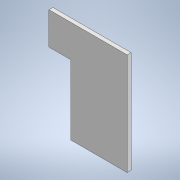
# Autodesk Inventor part: PCB_2_Miras
Saved by Autodesk Inventor 2022 (Build 260153000, 153)
## iProperties
Created: 2023-01-03
Part Number: PCB_2_Miras
Material: Generic
Document SubType Name: Modeling
Designer: Kamil
Density: 1 g/cm^3
Appearance: Default
Author: Kamil
Autodesk Inventor part; units mm, degrees
ref_plane "YZ Plane" through (0, 0, 0) normal (1, 0, 0) x (0, 1, 0)
ref_plane "XZ Plane" through (0, 0, 0) normal (0, 1, 0) x (-1, 0, 0)
ref_plane "XY Plane" through (0, 0, 0) normal (0, 0, 1) x (1, 0, 0)
sketch "Sketch1" plane through (0, 0, 0) normal (0, 0, 1) x (1, 0, 0)
  line L0 (12.5, -5.24) -> (15, -5.24) projected
  line L1 (15, -5.24) -> (15, -10.24) projected
  line L2 (15, -10.24) -> (12.5, -10.24) projected
  arc A0 (12.5, -5.24) -> (12.5, -10.24) centre (12.5, -7.74) ccw projected
  line L3 (-15, -5.24) -> (-12.5, -5.24) projected
  arc A1 (-12.5, -10.24) -> (-12.5, -5.24) centre (-12.5, -7.74) ccw projected
  line L4 (-12.5, -10.24) -> (-15, -10.24) projected
  line L5 (-15, -10.24) -> (-15, -5.24) projected
  circle A2 centre (-7.5, -12.2) radius 1.75 projected
  circle A3 centre (7.5, -12.2) radius 1.75 projected
  line L6 (37.5, 31.0066) -> (-37.5, 31.0066) projected
  line L7 (-37.5, 31.0066) -> (-37.5, -15.4) projected
  line L8 (-37.5, -15.4) -> (37.5, -15.4) projected
  line L9 (37.5, -15.4) -> (37.5, -10.4) projected
  line L10 (17.8602, 13.1005) -> (17.8602, -3.2) projected
  line L11 (17.8602, -3.2) -> (11.3436, -3.2) projected
  line L12 (11.3436, -3.2) -> (6.7283, -5.8186) projected
  line L13 (6.7283, -5.8186) -> (-6.7283, -5.8186) projected
  line L14 (-6.7283, -5.8186) -> (-11.3436, -3.2) projected
  line L15 (-11.3436, -3.2) -> (-17.8602, -3.2) projected
  line L16 (-17.8602, -3.2) -> (-17.8602, 13.1005) projected
  line L17 (-13.55, 13.1005) -> (-17.8602, 13.1005) projected
  line L18 (-13.55, 23.254) -> (-13.55, 13.1005) projected
  line L19 (2.4, 23.254) -> (-13.55, 23.254) projected
  line L20 (2.4, 25.954) -> (2.4, 23.254) projected
  line L21 (4, 25.954) -> (2.4, 25.954) projected
  line L22 (4, 23.254) -> (4, 25.954) projected
  line L23 (8.95, 23.254) -> (4, 23.254) projected
  line L24 (8.95, 13.1005) -> (8.95, 23.254) projected
  line L25 (17.8602, 13.1005) -> (8.95, 13.1005) projected
  line L26 (50, 22.6643) -> (44, 22.6643) projected
  line L27 (44, 22.6643) -> (44, -4.7413) projected
  arc A4 (44, -9.7413) -> (44, -4.7413) centre (44, -7.2413) ccw projected
  line L28 (44, -9.7413) -> (44, -18.8012) projected
  line L29 (44, -18.8012) -> (50, -18.8012) projected
  line L30 (50, -18.8012) -> (50, 22.6643) projected
  line L31 (40.2471, -8.6254) -> (44, -18.8012) projected
  line L32 (44, -9.7413) -> (44, -18.8012) projected
  arc A5 (44, -4.7413) -> (44, -9.7413) centre (44, -7.2413) ccw projected
  line L33 (44, 4.3187) -> (44, -4.7413) projected
  line L34 (44, 4.3187) -> (40.2471, -5.8572) projected
  arc A6 (40.2471, -5.8572) -> (40.2471, -8.6254) centre (44, -7.2413) ccw projected
  line L35 (8.95, 13.1005) -> (37.5, 13.1005)
  line L36 (37.5, 13.1005) -> (37.5, 31.0066)
  line L37 (37.5, 31.0066) -> (8.95, 31.0066)
  line L38 (8.95, 31.0066) -> (8.95, 13.1005)
  line L39 (44, 18.1772) -> (41, 18.1772)
  line L40 (41, 18.1772) -> (41, 7.8033)
  line L41 (41, 7.8033) -> (44, 7.8033)
  line L42 (44, 7.8033) -> (44, 18.1772)
  line L43 (37.5, 31.0066) -> (41, 31.0066)
  line L44 (41, 31.0066) -> (41, 1.9316)
  line L45 (41, 1.9316) -> (37.5, 1.9316)
  line L46 (37.5, 1.9316) -> (37.5, 31.0066)
  line L47 (8.95, 31.0066) -> (41, 31.0066)
  line L48 (41, 31.0066) -> (41, 23.254)
  line L49 (41, 23.254) -> (8.95, 23.254)
  line L50 (8.95, 23.254) -> (8.95, 31.0066)
  line L51 (17.8602, 13.1005) -> (37.5, 13.1005)
  line L52 (37.5, 13.1005) -> (37.5, -15.4)
  line L53 (37.5, -15.4) -> (17.8602, -15.4)
  line L54 (17.8602, -15.4) -> (17.8602, 13.1005)
  line L55 (37.5, -15.4) -> (41, -15.4)
  line L56 (41, -15.4) -> (41, 1.9316)
  line L57 (41, 1.9316) -> (37.5, 1.9316)
  line L58 (37.5, 1.9316) -> (37.5, -15.4)
  circle A7 centre (36, -10.4) radius 1.5 projected
  line L59 (37.5, -10.4) -> (37.5, 31.0066) projected
  arc A8 (-17.7252, -6.9095) -> (-17.704, -4.5096) centre (-17.7146, -5.7096) ccw projected
  line L60 (-17.7252, -6.9095) -> (-18.8252, -6.8998) projected
  arc A9 (-18.8039, -4.4999) -> (-18.8252, -6.8998) centre (-18.8145, -5.6998) ccw projected
  line L61 (-18.8039, -4.4999) -> (-17.704, -4.5096) projected
  circle A10 centre (21.3634, 8.1005) radius 1.5 projected
  arc A11 (-17.5172, 16.5895) -> (-17.496, 18.9894) centre (-17.5066, 17.7895) ccw projected
  line L62 (-17.5172, 16.5895) -> (-18.6172, 16.5993) projected
  arc A12 (-18.5959, 18.9992) -> (-18.6172, 16.5993) centre (-18.6065, 17.7992) ccw projected
  line L63 (-18.5959, 18.9992) -> (-17.496, 18.9894) projected
  point P0 (0, 0)
  point P1 (41, -3.8157)
  point P2 (8.95, 31.0066)
  point P3 (41, -10.6668)
  dimension "d0" = 3
  constraints: 48 end point, 12 parallel, 6 horizontal, 6 perpendicular, 2 point on line, 1 horizontal alignment
  measures "d0" distance of L41.end L40.end
extrude "Extrusion1" add sketch "Sketch1" along normal blind 3.1 contours L36 L49 L38 L6 | L43 L44 L49 L36 | L49 L44 L40 L45 L46 L36 | L36 L35 L25 L24 L49 | A7 | L46 L52 L9 L8 L54 L10 L35 | L45 L56 L34 A6 L31 L55 L9 L52 | A10
sketch "Sketch2" plane through (0, 0, 0) normal (0, 0, -1) x (-1, 0, 0)
  line L0 (-40.2471, -5.8572) -> (-41, -3.8157) projected
  arc A0 (-40.2471, -8.6254) -> (-40.2471, -5.8572) centre (-44, -7.2413) ccw projected
  line L1 (-41, -10.6668) -> (-40.2471, -8.6254) projected
  line L2 (-41, -15.4) -> (-41, -10.6668) projected
  line L3 (-17.8602, -15.4) -> (-41, -15.4) projected
  line L4 (-17.8602, 13.1005) -> (-17.8602, -15.4) projected
  line L5 (-8.95, 13.1005) -> (-17.8602, 13.1005) projected
  line L6 (-8.95, 31.0066) -> (-8.95, 13.1005) projected
  line L7 (-41, 31.0066) -> (-8.95, 31.0066) projected
  line L8 (-41, -3.8157) -> (-41, 31.0066) projected
  point P0 (0, 0)
extrude "Extrusion2" cut sketch "Sketch2" against normal blind 1.5
sketch "Sketch3" plane through (41, -3.8157, 3.1) normal (1, 0, 0) x (0, 0, -1)
  line L0 (24.6867, 44.1065) -> (27.0867, 44.1065) projected
  line L1 (27.0867, 44.1065) -> (27.0867, 31.3518) projected
  line L2 (27.0867, 31.3518) -> (24.6867, 31.3518) projected
  line L3 (24.6867, 31.3518) -> (24.6867, 44.1065) projected
  line L4 (36.2, 74.2694) -> (-3.9, 26.48) projected
  line L5 (-3.9, -14.9855) -> (-3.9, 26.48) projected
  line L6 (-3.9, -14.9855) -> (7.1, -14.9855) projected
  line L7 (7.1, -14.9855) -> (7.1, 1.1145) projected
  arc A0 (25.2, 19.2145) -> (7.1, 1.1145) centre (25.2, 1.1145) ccw projected
  line L8 (25.2, 19.2145) -> (36.2, 19.2145) projected
  line L9 (36.2, 19.2145) -> (36.2, 74.2694) projected
  line L10 (1.6, 0) -> (1.6, 34.8223) projected
  line L11 (1.6, 34.8223) -> (0, 34.8223) projected
  line L12 (0, 0) -> (0, 34.8223) projected
  line L13 (1.6, 0) -> (0, 0) projected
  line L14 (0, 0) -> (0, 34.8223) projected
  line L15 (0, 30.197) -> (1.6, 30.197)
  point P0 (3.1, 3.8157)
  constraints: 2 end point, 2 point on line, 1 perpendicular
extrude "Extrusion3" cut sketch "Sketch3" against normal through all contours L10 L15 L12 L4 | L4 L12 L11 L10
sketch "Sketch4" plane through (0, 0, 3.1) normal (0, 0, 1) x (1, 0, 0)
  line L0 (31.7, -15.7) -> (31.7, 9.3) projected
  line L1 (41, 26.3813) -> (8.95, 26.3813) projected
  line L2 (8.95, 26.3813) -> (8.95, 13.1005) projected
  line L3 (8.95, 13.1005) -> (17.8602, 13.1005) projected
  line L4 (17.8602, 13.1005) -> (17.8602, -15.4) projected
  line L5 (17.8602, -15.4) -> (41, -15.4) projected
  line L6 (41, -15.4) -> (41, -10.6668) projected
  line L7 (41, -10.6668) -> (40.2471, -8.6254) projected
  arc A0 (40.2471, -5.8572) -> (40.2471, -8.6254) centre (44, -7.2413) ccw projected
  line L8 (40.2471, -5.8572) -> (41, -3.8157) projected
  line L9 (41, -3.8157) -> (41, 26.3813) projected
  line L10 (41, -15.4) -> (41, -10.6668) projected
  line L11 (41, -3.8157) -> (41, -10.6668)
  point P0 (0, 0)
  constraints: 2 end point, 1 collinear
extrude "Extrusion4" add sketch "Sketch4" against normal blind 1.6 contours L11 L7 A0 L8
sketch "Sketch5" plane through (0, 0, 3.1) normal (0, 0, 1) x (1, 0, 0)
  line L0 (41, 26.3813) -> (8.95, 26.3813) projected
  line L1 (8.95, 26.3813) -> (8.95, 13.1005) projected
  line L2 (8.95, 13.1005) -> (17.8602, 13.1005) projected
  line L3 (17.8602, 13.1005) -> (17.8602, -15.4) projected
  line L4 (17.8602, -15.4) -> (41, -15.4) projected
  line L5 (41, -15.4) -> (41, 26.3813) projected
  line L6 (15, 8.3178) -> (15, -1.2725) projected
  line L7 (8.95, 13.1005) -> (17.8602, 13.1005) projected
  line L8 (17.8602, 13.1005) -> (16.3634, 13.1005)
  line L9 (16.3634, 13.1005) -> (16.3634, -15.4)
  line L10 (16.3634, -15.4) -> (17.8602, -15.4)
  line L11 (17.8602, -15.4) -> (17.8602, 13.1005)
  point P0 (0, 0)
  constraints: 8 end point, 2 parallel, 1 horizontal, 1 perpendicular
extrude "Extrusion5" add sketch "Sketch5" against normal blind 1.6 contours L10 L9 L2 L3
sketch "Sketch6" plane through (0, 0, 3.1) normal (0, 0, 1) x (1, 0, 0)
  line L0 (41, 26.3813) -> (8.95, 26.3813) projected
  line L1 (8.95, 26.3813) -> (8.95, 13.1005) projected
  line L2 (8.95, 13.1005) -> (16.3634, 13.1005) projected
  line L3 (16.3634, 13.1005) -> (16.3634, -15.4) projected
  line L4 (16.3634, -15.4) -> (41, -15.4) projected
  line L5 (41, -15.4) -> (41, 26.3813) projected
  line L6 (16.3634, -15.4) -> (41, -15.4) projected
  line L7 (28.6817, -15.4) -> (28.6817, 26.3813)
  line L8 (41, 26.3813) -> (8.95, 26.3813) projected
  line L9 (28.6817, -15.4) -> (28.6817, -9.9)
  line L10 (28.6817, 26.3813) -> (28.6817, 20.8813)
  line L11 (16.3634, 13.1005) -> (41, 13.1005)
  line L12 (41, -15.4) -> (41, 26.3813) projected
  line L13 (16.3634, 13.1005) -> (21.3634, 13.1005)
  line L14 (21.3634, 13.1005) -> (21.3634, 8.1005)
  line L15 (21.3634, 8.1005) -> (16.3634, 8.1005)
  line L16 (16.3634, 8.1005) -> (16.3634, 13.1005)
  line L17 (41, -15.4) -> (36, -15.4)
  line L18 (36, -15.4) -> (36, -10.4)
  line L19 (36, -10.4) -> (41, -10.4)
  line L20 (41, -10.4) -> (41, -15.4)
  circle A0 centre (21.3634, 8.1005) radius 1.5
  circle A1 centre (36, -10.4) radius 1.5
  point P0 (0, 0)
  dimension "d11" = 5.5
  dimension "d12" = 5.5
  dimension "d13" = 5
  dimension "d14" = 5
  dimension "d15" = 5
  dimension "d16" = 5
  dimension "d17" = 3
  dimension "d18" = 3
  constraints: 24 end point, 4 parallel, 4 perpendicular, 4 point on line, 2 centre point, 2 coincident, 2 horizontal, 1 midpoint
  measures "d11" distance of L7.start L9.end
  measures "d12" distance of L7.end L10.end
  measures "d13" distance of L14.end L15.end
  measures "d14" distance of L13.end L14.end
  measures "d15" distance of L18.end L19.end
  measures "d16" distance of L17.end L18.end
  measures "d17" diameter of A0
  measures "d18" diameter of A1
extrude "Extrusion6" cut sketch "Sketch6" against normal blind 1.6 contours A1 L18 L19 | L19 L18 A1 | A0 L15 L14 | L14 L15 A0
body "Solid1"
